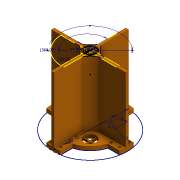
# Autodesk Inventor part: SunTrackerHolder
Saved by Autodesk Inventor 2020.3 (Build 243373000, 373)
## iProperties
Created: 2020-12-01
Part Number: SunTrackerHolder
Material: Generic
Document SubType Name: Modeling
Designer: Yusuf
Mass: 46.1078 g
Surface Area: 327.015 cm^2
Volume: 46.1078 cm^3
Density: 1 g/cm^3
Appearance: Orange
Author: Yusuf
Autodesk Inventor part; units mm, degrees
ref_plane "YZ Plane" through (0, 0, 0) normal (1, 0, 0) x (0, 1, 0)
ref_plane "XZ Plane" through (0, 0, 0) normal (0, 1, 0) x (-1, 0, 0)
ref_plane "XY Plane" through (0, 0, 0) normal (0, 0, 1) x (1, 0, 0)
sketch "Sketch1" plane through (0, 0, 0) normal (0, 1, 0) x (-1, 0, 0)
  circle A0 centre (0, 0) radius 30
  dimension "d0" = 60
  constraints: 1 centre point, 1 coincident
  measures "d0" diameter of A0
extrude "Extrusion1" add sketch "Sketch1" along normal blind 4
sketch "Sketch2" plane through (0, 4, 0) normal (0, 1, 0) x (1, 0, 0)
  circle A0 centre (0, 0) radius 30 projected
  line L0 (-29.9625, -1.5) -> (-1.5, -1.5)
  line L1 (1.5, -1.5) -> (29.9625, -1.5)
  line L2 (29.9625, 1.5) -> (1.5, 1.5)
  line L3 (-1.5, 1.5) -> (-29.9625, 1.5)
  line L4 (-1.5, 29.9625) -> (-1.5, 1.5)
  line L5 (-1.5, -1.5) -> (-1.5, -29.9625)
  line L6 (1.5, -29.9625) -> (1.5, -1.5)
  line L7 (1.5, 1.5) -> (1.5, 29.9625)
  point P0 (-29.9625, 0)
  point P1 (0, 29.9625)
  point P2 (-1.5, 0)
  dimension "d5" = 3
  dimension "d6" = 3
  dimension "d7" = 3
  dimension "d8" = 3
  constraints: 16 end point, 8 parallel, 3 point on circle, 2 horizontal, 2 horizontal alignment, 1 vertical alignment
  measures "d5" distance between parallel lines of L2 L1
  measures "d6" distance between parallel lines of L7 L4
  measures "d7" distance between parallel lines of L3 L0
  measures "d8" distance between parallel lines of L6 L5
extrude "Extrusion2" add sketch "Sketch2" along normal blind 70 contours A0 L1 L6 L5 L0 L3 L4 L7 L2
sketch "Sketch5" plane through (0, 4, 0) normal (0, 1, 0) x (1, 0, 0)
  circle A0 centre (12.5637, 12.5637) radius 6.5
  line L0 (29.9625, 1.5) -> (1.5, 1.5) projected
  line L1 (1.5, 1.5) -> (1.5, 29.9625) projected
  line L2 (12.5637, 12.5637) -> (1.5, 12.5637) construction
  line L3 (12.5637, 12.5637) -> (12.5637, 1.5) construction
  line L4 (16.5637, 12.5637) -> (8.5637, 12.5637) construction
  line L5 (11.8526, 19.0247) -> (11.8526, 6.1027)
  line L6 (13.3526, 6.1117) -> (13.3526, 19.0157)
  line L7 (19.0195, 11.807) -> (6.1079, 11.807)
  line L8 (19.0211, 13.307) -> (6.1063, 13.307)
  point P0 (0, 0)
  point P1 (12.5637, 7.0319)
  point P2 (13.3526, 11.807)
  point P3 (13.3526, 13.307)
  point P4 (11.8526, 13.307)
  point P5 (11.8526, 11.807)
  dimension "d20" = 13
  dimension "d25" = 8
  dimension "d58" = 1.5
  dimension "d59" = 1.5
  constraints: 14 end point, 3 perpendicular, 3 point on line, 2 horizontal, 2 midpoint, 1 horizontal alignment, 1 parallel, 1 vertical, 1 vertical alignment, 10 other
  measures "d25" distance of L4.end L4.start
  measures "d58" distance between parallel lines of L6 L5
  measures "d59" distance between parallel lines of L8 L7
extrude "Extrusion5" cut sketch "Sketch5" against normal blind 2
extrude "Extrusion6" cut sketch "Sketch5" against normal up to surface (4 mm away) contours L8 L6 A0 | A0 L6 L7 | L5 L8 A0 | A0 L7 L5
pattern_circular "Circular Pattern1" count 4 over 360 about axis through (0, -10, 0) along (0, 1, 0) of "Extrusion6", "Extrusion5"
sketch "Sketch8" plane through (0, 74, 0) normal (0, 1, 0) x (1, 0, 0)
  circle A0 centre (0, 0) radius 6.5
  circle A1 centre (0, 0) radius 5.5
  line L0 (-0.75, -5.4486) -> (-0.75, 5.4486)
  line L1 (-1.5, -29.9625) -> (-1.5, -1.5) projected
  line L2 (0.75, -5.4486) -> (0.75, 5.4486)
  line L3 (1.5, -1.5) -> (1.5, -29.9625) projected
  line L4 (-0.75, -3.138) -> (0.75, -3.138) construction
  arc A2 (-1.5, -10.2121) -> (-10.2121, -1.5) centre (-22.7442, -22.7442) ccw
  line L5 (0, 0) -> (-25.6194, -25.6194) construction
  arc A3 (-29.9625, -1.5) -> (-1.5, -29.9625) centre (0, 0) ccw projected
  line L6 (-1.5, -1.5) -> (-29.9625, -1.5) projected
  line L7 (-29.9625, -1.5) -> (-1.5, -1.5) projected
  arc A4 (10.2121, -1.5) -> (1.5, -10.2121) centre (22.7442, -22.7442) ccw
  arc A5 (1.5, 10.2121) -> (10.2121, 1.5) centre (22.7442, 22.7442) ccw
  arc A6 (-10.2121, 1.5) -> (-1.5, 10.2121) centre (-22.7442, 22.7442) ccw
  line L8 (-1.5, 29.9625) -> (-1.5, 1.5) projected
  line L9 (1.5, -1.5) -> (29.9625, -1.5) projected
  line L10 (29.9625, 1.5) -> (1.5, 1.5) projected
  line L11 (10.2121, 1.5) -> (13.7073, 1.5)
  line L12 (10.2121, -1.5) -> (13.7073, -1.5)
  line L13 (-10.2121, -1.5) -> (-14.8678, -1.5)
  line L14 (-10.2121, 1.5) -> (-14.8678, 1.5)
  point P0 (0, -3.138)
  point P1 (-10.2121, -1.5)
  point P2 (-1.5, -5.2915)
  point P3 (-5.2915, -1.5)
  dimension "d85" = 13
  dimension "d86" = 11
  dimension "d87" = 1.5
  dimension "d88" = 24.6651
  dimension "d89" = 45
  dimension "d92" = 360
  constraints: 16 end point, 12 point on circle, 8 point on line, 6 centre point, 2 parallel, 1 coincident, 1 horizontal, 1 midpoint, 1 perpendicular, 1 vertical alignment, 17 other
  measures "d85" diameter of A0
  measures "d86" diameter of A1
  measures "d87" distance between parallel lines of L2 L0
  measures "d88" radius of A2
  measures "d89" angle of L1 L5
extrude "Extrusion13" cut sketch "Sketch8" against normal up to surface (74 mm away) contours A1 L9 L3 L2 | A1 L3 L9 | A1 L0 L1 L6 | L6 L1 A1
extrude "Extrusion14" add sketch "Sketch8" against normal up to surface (74 mm away) contours L6 A1 L1 A0 | A0 L1 A2 L6
pattern_circular "Circular Pattern3" count 4 over 360 about axis through (0, -10, 0) along (0, 1, 0) of "Extrusion14"
extrude "Extrusion15" cut sketch "Sketch8" against normal blind 2 contours A0 L9 A1 L10 | L10 A1 L8 A0 | A0 L3 A1 L9 | L8 A1 L6 A0 | A1 L9 L3 L2 | A0 L1 A1 L3 | A1 L3 L9 | L6 A1 L1 A0 | A1 L0 L1 L6 | L2 A1 L0 | L6 L1 A1
sketch "Sketch10" plane through (0, 0, 0) normal (0, 1, 0) x (-1, 0, 0)
  circle A0 centre (0, 0) radius 27.5
  circle A1 centre (0, 0) radius 40
  line L0 (10.2121, 1.5) -> (29.9625, 1.5) projected
  line L1 (25.2159, 1.5) -> (39.9719, 1.5)
  line L2 (29.9625, -1.5) -> (10.2121, -1.5) projected
  line L3 (25.2159, -1.5) -> (39.9719, -1.5)
  line L4 (25.2159, -1.5) -> (25.2159, 1.5)
  point P0 (27.4591, 1.5)
  point P1 (27.4591, -1.5)
  dimension "d106" = 55
  dimension "d107" = 80
  constraints: 6 end point, 2 centre point, 2 coincident, 2 collinear, 2 point on circle, 2 point on line, 1 perpendicular
  measures "d106" diameter of A0
  measures "d107" diameter of A1
extrude "Extrusion17" add sketch "Sketch10" along normal up to surface (4 mm away) contours A0 L0 L1 A1 L3 L2 | A0 L2 L3 A1 L1 L0
extrude "Extrusion18" add sketch "Sketch10" along normal up to surface (74 mm away) contours A0 L0 L1 A1 L3 L2 picked at (33.3083, 0)
sketch "Sketch11" plane through (0, 4, 0) normal (0, 1, 0) x (1, 0, 0)
  circle A0 centre (0, 0) radius 40 projected
  line L0 (-39.2906, -7.5) -> (-26.4575, -7.5)
  line L1 (-10.2121, -1.5) -> (-29.9625, -1.5) projected
  circle A1 centre (-36, -4.5) radius 1.5
  circle A2 centre (0, 0) radius 27.5 projected
  line L2 (-7.5, -3.3264) -> (-7.5, -39.2906)
  line L3 (-26.4575, -7.5) -> (-7.5, -7.5)
  circle A3 centre (-4.5, -36) radius 1.5
  circle A4 centre (-27.1293, -4.5) radius 1.5
  circle A5 centre (-4.5, -27.1293) radius 1.5
  point P0 (-7.5, -26.4575)
  dimension "d112" = 6
  dimension "d113" = 3
  dimension "d114" = 7.5
  dimension "d115" = 3
  dimension "d116" = 36
  dimension "d117" = 36
  dimension "d118" = 3
  dimension "d119" = 3
  dimension "d125" = 3
  constraints: 6 end point, 6 point on circle, 4 centre point, 2 point on line, 1 equal radius, 1 horizontal, 1 horizontal alignment, 1 perpendicular, 1 vertical, 1 vertical alignment
  measures "d112" distance between parallel lines of L0 L1
  measures "d113" diameter of A1
  measures "d114" distance from line of L2 point (0, 0)
  measures "d115" diameter of A3
  measures "d116" horizontal distance of A2.centre A1.centre
  measures "d117" vertical distance of A2.centre A3.centre
  measures "d118" distance from line of L0 A1.centre
  measures "d119" distance from line of L2 A3.centre
  measures "d125" diameter of A5
extrude "Extrusion19" cut sketch "Sketch11" against normal up to surface (4 mm away) contours L0 A2 L2 A0 | A4 A2 | A2 A4 | A5 A2 | A2 A5 | A1 | A3
pattern_circular "Circular Pattern4" count 4 over 360 about axis through (0, -10, 0) along (0, 1, 0) of "Extrusion18", "Extrusion19"
sketch "Sketch12" plane through (0, 0, 0) normal (0, -1, 0) x (1, 0, 0)
  line L0 (26.4575, 7.5) -> (39.2906, 7.5) projected
  line L1 (39.0223, 7.5) -> (26.4575, 7.5)
  arc A0 (7.5, 39.2906) -> (-7.5, 39.2906) centre (0, 0) ccw projected
  line L2 (7.5, 39.2906) -> (7.5, 26.4575) projected
  line L3 (7.5, 39.2906) -> (7.5, 26.4575)
  constraints: 4 end point, 1 collinear, 1 horizontal
equation "\"d94\" = d85"
body "Solid1"
